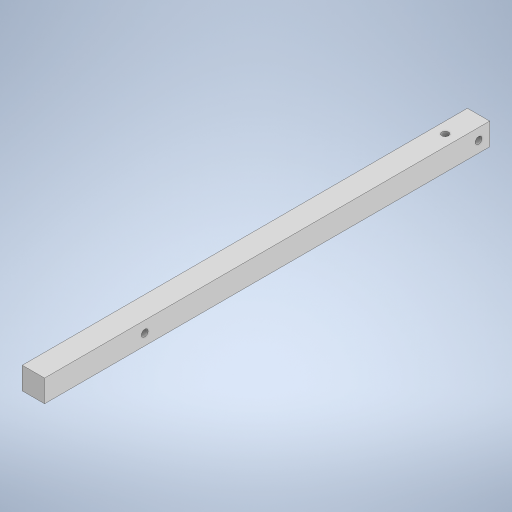
# Autodesk Inventor part: Dai
Saved by Autodesk Inventor 2023 (Build 270158000, 158)
## iProperties
Created: 2022-10-24
Part Number: Dai
Material: 一般
Document SubType Name: Modeling
Designer: banru
Density: 1 g/cm^3
Appearance: 既定
Author: banru
Autodesk Inventor part; units mm, degrees
ref_plane "YZ Plane" through (0, 0, 0) normal (1, 0, 0) x (0, 1, 0)
ref_plane "XZ Plane" through (0, 0, 0) normal (0, 1, 0) x (-1, 0, 0)
ref_plane "XY Plane" through (0, 0, 0) normal (0, 0, 1) x (1, 0, 0)
sketch "スケッチ1" plane through (0, 0, 0) normal (1, 0, 0) x (0, 1, 0)
  line L0 (0, 0) -> (10, 0)
  line L1 (10, 0) -> (10, -200)
  line L2 (10, -200) -> (0, -200)
  line L3 (0, -200) -> (0, 0)
  dimension "d0" = 10
  dimension "d1" = 200
  constraints: 8 end point, 2 parallel, 1 horizontal, 1 perpendicular
  measures "d0" distance of L1.end L2.end
  measures "d1" distance of L0.end L1.end
extrude "押し出し1" add sketch "スケッチ1" along normal blind 10
sketch "スケッチ2" plane through (10, 0, 0) normal (1, 0, 0) x (0, 0, -1)
  line L0 (200, 0) -> (200, 10) projected
  line L1 (0, 10) -> (0, 0) projected
  point P0 (195, 5)
  point P1 (45, 5)
  point P2 (200, 5)
  point P3 (200, 5)
  point P4 (200, 5)
  point P5 (0, 5)
  dimension "d4" = 5
  dimension "d5" = 45
  constraints: 4 midpoint, 2 horizontal alignment
  measures "d4" distance of point (200, 5) point (195, 5)
  measures "d5" distance of point (0, 5) point (45, 5)
hole "穴1" at (10, 5, -195) at (10, 5, -45) direction (-1, 0, 0) diameter 3.1 end through all
sketch "スケッチ3" plane through (0, 10, 0) normal (0, 1, 0) x (1, 0, 0)
  line L0 (0, 200) -> (10, 200) projected
  point P0 (0, 0)
  point P1 (5, 185)
  point P2 (5, 200)
  point P3 (5, 200)
  dimension "d13" = 15
  constraints: 2 midpoint, 1 vertical alignment
  measures "d13" distance of point (5, 185) point (5, 200)
hole "穴2" at (5, 10, -185) direction (0, -1, 0) diameter 3.1 end through all
